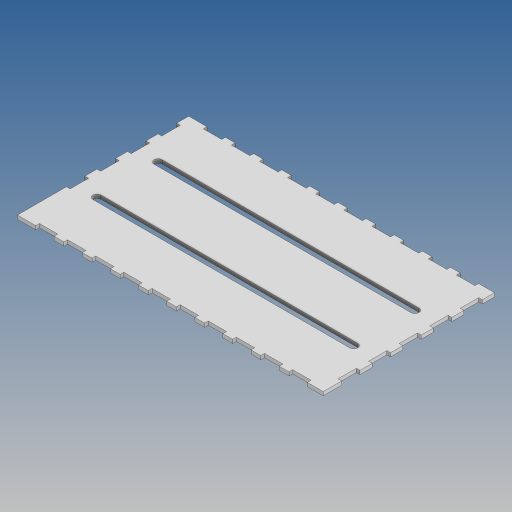
# Autodesk Inventor part: Pieza1
Saved by Autodesk Inventor 2024 (Build 280153000, 153)
## iProperties
Created: 2024-05-31
Part Number: Pieza1
Material: Genérico
Document SubType Name: Modeling
Designer: Pablo
Density: 1 g/cm^3
Appearance: Valor por defecto
Author: Pablo
Autodesk Inventor part; units mm, degrees
ref_plane "YZ Plane" through (0, 0, 0) normal (1, 0, 0) x (0, 1, 0)
ref_plane "XZ Plane" through (0, 0, 0) normal (0, 1, 0) x (-1, 0, 0)
ref_plane "XY Plane" through (0, 0, 0) normal (0, 0, 1) x (1, 0, 0)
sketch "Boceto1" plane through (0, 0, 0) normal (0, 1, 0) x (-1, 0, 0)
  line L0 (0, 0) -> (250, 0)
  line L1 (250, 0) -> (250, -140)
  line L2 (250, -140) -> (0, -140)
  line L3 (0, -140) -> (0, 0)
  line L4 (250, -15) -> (247, -15)
  line L5 (247, -15) -> (247, -30)
  line L6 (247, -30) -> (250, -30)
  line L7 (250, -30) -> (250, -15)
  line L8 (125, 0) -> (125, -140) construction
  line L9 (250, -70) -> (0, -70) construction
  line L10 (250, -40) -> (247, -40)
  line L11 (247, -40) -> (247, -55)
  line L12 (247, -55) -> (250, -55)
  line L13 (250, -55) -> (250, -40)
  line L14 (250, -65) -> (247, -65)
  line L15 (247, -65) -> (247, -80)
  line L16 (247, -80) -> (250, -80)
  line L17 (250, -80) -> (250, -65)
  line L18 (250, -90) -> (247, -90)
  line L19 (247, -90) -> (247, -105)
  line L20 (247, -105) -> (250, -105)
  line L21 (250, -105) -> (250, -90)
  line L22 (250, -115) -> (247, -115)
  line L23 (247, -115) -> (247, -130)
  line L24 (247, -130) -> (250, -130)
  line L25 (250, -130) -> (250, -115)
  line L26 (235, 0) -> (220, 0)
  line L27 (220, 0) -> (220, -3)
  line L28 (220, -3) -> (235, -3)
  line L29 (235, -3) -> (235, 0)
  line L30 (197, -3) -> (212, -3)
  line L31 (212, -3) -> (212, 0)
  line L32 (212, 0) -> (197, 0)
  line L33 (197, 0) -> (197, -3)
  line L34 (174, -3) -> (189, -3)
  line L35 (189, -3) -> (189, 0)
  line L36 (189, 0) -> (174, 0)
  line L37 (174, 0) -> (174, -3)
  line L38 (151, -3) -> (166, -3)
  line L39 (166, -3) -> (166, 0)
  line L40 (166, 0) -> (151, 0)
  line L41 (151, 0) -> (151, -3)
  line L42 (128, -3) -> (143, -3)
  line L43 (143, -3) -> (143, 0)
  line L44 (143, 0) -> (128, 0)
  line L45 (128, 0) -> (128, -3)
  line L46 (105, -3) -> (120, -3)
  line L47 (120, -3) -> (120, 0)
  line L48 (120, 0) -> (105, 0)
  line L49 (105, 0) -> (105, -3)
  line L50 (82, -3) -> (97, -3)
  line L51 (97, -3) -> (97, 0)
  line L52 (97, 0) -> (82, 0)
  line L53 (82, 0) -> (82, -3)
  line L54 (59, -3) -> (74, -3)
  line L55 (74, -3) -> (74, 0)
  line L56 (74, 0) -> (59, 0)
  line L57 (59, 0) -> (59, -3)
  line L58 (36, -3) -> (51, -3)
  line L59 (51, -3) -> (51, 0)
  line L60 (51, 0) -> (36, 0)
  line L61 (36, 0) -> (36, -3)
  line L62 (13, -3) -> (28, -3)
  line L63 (28, -3) -> (28, 0)
  line L64 (28, 0) -> (13, 0)
  line L65 (13, 0) -> (13, -3)
  line L66 (235, -140) -> (220, -140)
  line L67 (220, -140) -> (220, -137)
  line L68 (220, -137) -> (235, -137)
  line L69 (235, -137) -> (235, -140)
  line L70 (197, -137) -> (212, -137)
  line L71 (212, -137) -> (212, -140)
  line L72 (212, -140) -> (197, -140)
  line L73 (197, -140) -> (197, -137)
  line L74 (174, -137) -> (189, -137)
  line L75 (189, -137) -> (189, -140)
  line L76 (189, -140) -> (174, -140)
  line L77 (174, -140) -> (174, -137)
  line L78 (151, -137) -> (166, -137)
  line L79 (166, -137) -> (166, -140)
  line L80 (166, -140) -> (151, -140)
  line L81 (151, -140) -> (151, -137)
  line L82 (128, -137) -> (143, -137)
  line L83 (143, -137) -> (143, -140)
  line L84 (143, -140) -> (128, -140)
  line L85 (128, -140) -> (128, -137)
  line L86 (105, -137) -> (120, -137)
  line L87 (120, -137) -> (120, -140)
  line L88 (120, -140) -> (105, -140)
  line L89 (105, -140) -> (105, -137)
  line L90 (82, -137) -> (97, -137)
  line L91 (97, -137) -> (97, -140)
  line L92 (97, -140) -> (82, -140)
  line L93 (82, -140) -> (82, -137)
  line L94 (59, -137) -> (74, -137)
  line L95 (74, -137) -> (74, -140)
  line L96 (74, -140) -> (59, -140)
  line L97 (59, -140) -> (59, -137)
  line L98 (36, -137) -> (51, -137)
  line L99 (51, -137) -> (51, -140)
  line L100 (51, -140) -> (36, -140)
  line L101 (36, -140) -> (36, -137)
  line L102 (13, -137) -> (28, -137)
  line L103 (28, -137) -> (28, -140)
  line L104 (28, -140) -> (13, -140)
  line L105 (13, -140) -> (13, -137)
  line L106 (0, -15) -> (3, -15)
  line L107 (3, -15) -> (3, -30)
  line L108 (3, -30) -> (0, -30)
  line L109 (0, -30) -> (0, -15)
  line L110 (0, -40) -> (3, -40)
  line L111 (3, -40) -> (3, -55)
  line L112 (3, -55) -> (0, -55)
  line L113 (0, -55) -> (0, -40)
  line L114 (0, -65) -> (3, -65)
  line L115 (3, -65) -> (3, -80)
  line L116 (3, -80) -> (0, -80)
  line L117 (0, -80) -> (0, -65)
  line L118 (0, -90) -> (3, -90)
  line L119 (3, -90) -> (3, -105)
  line L120 (3, -105) -> (0, -105)
  line L121 (0, -105) -> (0, -90)
  line L122 (0, -115) -> (3, -115)
  line L123 (3, -115) -> (3, -130)
  line L124 (3, -130) -> (0, -130)
  line L125 (0, -130) -> (0, -115)
  line L126 (20, -45) -> (230, -45) construction
  line L127 (20, -48.25) -> (230, -48.25)
  line L128 (230, -41.75) -> (20, -41.75)
  arc A0 (20, -41.75) -> (20, -48.25) centre (20, -45) ccw
  arc A1 (230, -48.25) -> (230, -41.75) centre (230, -45) ccw
  line L129 (20, -95) -> (230, -95) construction
  line L130 (20, -98.25) -> (230, -98.25)
  line L131 (230, -91.75) -> (20, -91.75)
  arc A2 (20, -91.75) -> (20, -98.25) centre (20, -95) ccw
  arc A3 (230, -98.25) -> (230, -91.75) centre (230, -95) ccw
  line L132 (112.5, -20) -> (137.5, -20)
  line L133 (137.5, -20) -> (137.5, -120)
  line L134 (137.5, -120) -> (112.5, -120)
  line L135 (112.5, -120) -> (112.5, -20)
  line L136 (112.5, -20) -> (137.5, -120) construction
  line L137 (137.5, -20) -> (112.5, -120) construction
  point P0 (248.5, -15)
  point P1 (248.5, -40)
  point P2 (248.5, -65)
  point P3 (248.5, -90)
  point P4 (248.5, -115)
  point P5 (235, -1.5)
  point P6 (212, -1.5)
  point P7 (189, -1.5)
  point P8 (166, -1.5)
  point P9 (143, -1.5)
  point P10 (120, -1.5)
  point P11 (97, -1.5)
  point P12 (74, -1.5)
  point P13 (51, -1.5)
  point P14 (28, -1.5)
  point P15 (235, -138.5)
  point P16 (212, -138.5)
  point P17 (189, -138.5)
  point P18 (166, -138.5)
  point P19 (143, -138.5)
  point P20 (120, -138.5)
  point P21 (97, -138.5)
  point P22 (74, -138.5)
  point P23 (51, -138.5)
  point P24 (28, -138.5)
  point P25 (1.5, -15)
  point P26 (1.5, -40)
  point P27 (1.5, -65)
  point P28 (1.5, -90)
  point P29 (1.5, -115)
  point P30 (220, 0)
  point P31 (212, 0)
  point P32 (197, 0)
  point P33 (189, 0)
  point P34 (174, 0)
  point P35 (166, 0)
  point P36 (151, 0)
  point P37 (143, 0)
  point P38 (128, 0)
  point P39 (120, 0)
  point P40 (105, 0)
  point P41 (97, 0)
  point P42 (82, 0)
  point P43 (74, 0)
  point P44 (59, 0)
  point P45 (51, 0)
  point P46 (36, 0)
  point P47 (28, 0)
  point P48 (13, 0)
  point P49 (13, -140)
  point P50 (28, -140)
  point P51 (51, -140)
  point P52 (59, -140)
  point P53 (74, -140)
  point P54 (82, -140)
  point P55 (97, -140)
  point P56 (105, -140)
  point P57 (120, -140)
  point P58 (128, -140)
  point P59 (143, -140)
  point P60 (151, -140)
  point P61 (166, -140)
  point P62 (174, -140)
  point P63 (189, -140)
  point P64 (212, -140)
  point P65 (220, -140)
  point P66 (235, -140)
  point P67 (250, -130)
  point P68 (250, -105)
  point P69 (250, -80)
  point P70 (250, -55)
  point P71 (250, -30)
  point P72 (125, -45)
  point P73 (125, -95)
  point P74 (125, -70)
  point P75 (125, -70)
  dimension "d0" = 250
  dimension "d1" = 140
  dimension "d2" = 3
  dimension "d3" = 15
  dimension "d4" = 15
  dimension "d7" = 25
  dimension "d12" = 15
  dimension "d13" = 3
  dimension "d14" = 15
  dimension "d17" = 23
  dimension "d24" = 25
  dimension "d25" = 25
  dimension "d26" = 105
  dimension "d27" = 6.5
  dimension "d28" = 105
  dimension "d29" = 6.5
  dimension "d30" = 25
  dimension "d31" = 100
  constraints: 276 end point, 75 symmetric about line, 45 horizontal alignment, 28 parallel, 18 collinear, 10 midpoint, 8 point on circle, 8 tangent, 4 centre point, 4 perpendicular, 3 horizontal, 3 point on line, 2 vertical, 45 other
  measures "d0" distance of L1.end L3.start
  measures "d1" distance of L1.start L1.end
  measures "d2" distance of L6.end L5.end
  measures "d3" distance of L5.end L4.end
  measures "d7" distance of L4.start L10.start
  measures "d12" distance of L28.end L27.end
  measures "d13" distance of L27.end L26.end
  measures "d14" distance from line of point (235, -1.5) L1
  measures "d17" distance of L28.end L30.end
  measures "d24" distance of point (125, -45) point (125, -70)
  measures "d25" distance of point (125, -70) point (125, -95)
  measures "d26" distance of point (125, -45) L126.end
  measures "d27" diameter of A1
  measures "d28" distance of point (125, -95) L129.end
  measures "d29" diameter of A3
  measures "d30" distance of L133.end L134.end
  measures "d31" distance of L132.end L133.end
extrude "Extrusión1" add sketch "Boceto1" along normal blind 3 contours L0 L65 L62 L63 L61 L58 L59 L57 L54 L55 L53 L50 L51 L49 L46 L47 L45 L42 L43 L41 L38 L39 L37 L34 L35 L33 L30 L31 L27 L28 L29 L1 L4 L5 L6 L10 L11 L12 L14 L15 L16 L18 L19 L20 L22 L23 L24 L2 L69 L68 L67 L71 L70 L73 L75 L74 L77 L79 L78 L81 L83 L82 L85 L87 L86 L89 L91 L90 L93 L95 L94 L97 L99 L98 L101 L103 L102 L105 L3 L124 L123 L122 L120 L119 L118 L116 L115 L114 L112 L111 L110 L108 L107 L106 | L1 L6 L5 L4 | L127 L133 L131 L135 | L135 L132 L133 L128 | L130 L133 L134 L135
